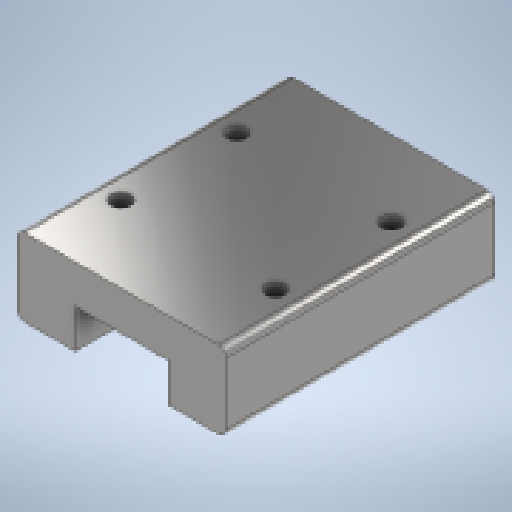
# Autodesk Inventor part: MGN12C Cart
Saved by Autodesk Inventor 2026.2 (Build 302298010, 298A)
## iProperties
Created: 2026-04-28
Part Number: MGN12C Cart
Material: Steel, Carbon
Document SubType Name: Modeling
Designer: chanh
Density: 7.85 g/cm^3
Appearance: Semi-Polished
Author: chanh
Autodesk Inventor part; units mm, degrees
ref_plane "YZ Plane" through (0, 0, 0) normal (1, 0, 0) x (0, 1, 0)
ref_plane "XZ Plane" through (0, 0, 0) normal (0, 1, 0) x (-1, 0, 0)
ref_plane "XY Plane" through (0, 0, 0) normal (0, 0, 1) x (1, 0, 0)
sketch "Sketch1" plane through (0, 0, 0) normal (0, 0, 1) x (1, 0, 0)
  line L0 (-6, 5) -> (6, 5)
  line L1 (6, 5) -> (6, 0)
  line L2 (6, 0) -> (-6, 0)
  line L3 (-6, 0) -> (-6, 5)
  line L4 (-6, 5) -> (6, 0) construction
  line L5 (6, 5) -> (-6, 0) construction
  line L6 (-13.5, 10) -> (13.5, 10)
  line L7 (13.5, 10) -> (13.5, 0)
  line L8 (13.5, 0) -> (-13.5, 0)
  line L9 (-13.5, 0) -> (-13.5, 10)
  line L10 (-13.5, 10) -> (13.5, 0) construction
  line L11 (13.5, 10) -> (-13.5, 0) construction
  point P0 (0, 0)
  point P1 (0, 2.5)
  point P2 (0, 0)
  point P3 (0, 5)
  point P4 (6, 0)
  point P5 (-6, 0)
  dimension "d0" = 12
  dimension "d1" = 5
  dimension "d2" = 27
  dimension "d3" = 10
  constraints: 24 end point, 6 midpoint, 4 parallel, 2 horizontal, 2 perpendicular, 1 coincident
  measures "d0" distance of L0.start L0.end
  measures "d1" distance of L0.end L1.end
  measures "d2" distance of L7.end L8.end
  measures "d3" distance of L6.end L7.end
extrude "Extrusion1" add sketch "Sketch1" along normal mid plane 34.7 contours L3 L8 L9 L6 L7 L1 L0
sketch "Sketch2" plane through (-13.5, 10, 17.35) normal (0, 1, 0) x (1, 0, 0)
  line L0 (23.5, 9.85) -> (3.5, 9.85) construction
  line L1 (3.5, 9.85) -> (3.5, 24.85) construction
  line L2 (3.5, 24.85) -> (23.5, 24.85) construction
  line L3 (23.5, 24.85) -> (23.5, 9.85) construction
  line L4 (23.5, 9.85) -> (3.5, 24.85) construction
  line L5 (3.5, 9.85) -> (23.5, 24.85) construction
  point P0 (13.5, 17.35)
  dimension "d6" = 20
  dimension "d7" = 15
  constraints: 12 end point, 4 coincident, 2 midpoint, 2 parallel, 1 horizontal, 1 perpendicular
  measures "d6" distance of L1.end L2.end
  measures "d7" distance of L0.end L1.end
hole "Hole1" at (-10, 10, 7.5) at (10, 10, 7.5) at (10, 10, -7.5) at (-10, 10, -7.5) direction (0, -1, 0) diameter 2.459 depth 4 thread size "M3x0.5" class "6H" standard "ISO Metric profile"
fillet "Fillet1" radius 1 4 edges at (13.5, 10, 0) (-13.5, 10, 0) (13.5, 0, 0) (-13.5, 0, 0)
body "Solid1"
